Autodesk Inventor part; units mm, degrees
(part 2 of 2)
sketch "Boceto5" plane through (0, 0, 0) normal (0, 0, 1) x (1, 0, 0)
  line L0 (-116.2875, 14.8964) -> (-116.2875, 0.0237) projected
  line L1 (-116.2875, 7.46) -> (97.4125, 7.46) construction
  line L2 (97.4125, 0.0237) -> (97.4125, 14.8964) projected
  line L3 (88.5625, 9.96) -> (-107.4375, 9.96) projected
  line L4 (88.6375, 9.8301) -> (88.5625, 9.96) projected
  line L5 (-107.5125, 5.09) -> (-107.4375, 4.96) projected
  line L6 (-107.4375, 4.96) -> (88.5625, 4.96) projected
  line L7 (88.5625, 4.96) -> (88.6375, 5.09) projected
  line L8 (88.6375, 5.09) -> (97.4125, 0.0237) projected
  line L9 (97.4125, 0.0237) -> (97.4125, 14.8964) projected
  line L10 (97.4125, 14.8964) -> (88.6375, 9.8301) projected
  line L11 (88.6375, 9.8301) -> (88.5625, 9.96) projected
  line L12 (88.5625, 9.96) -> (-107.4375, 9.96) projected
  line L13 (-107.4375, 9.96) -> (-107.5125, 9.8301) projected
  line L14 (-107.5125, 9.8301) -> (-116.2875, 14.8964) projected
  line L15 (-116.2875, 14.8964) -> (-116.2875, 0.0237) projected
  line L16 (-116.2875, 0.0237) -> (-107.5125, 5.09) projected
  line L17 (88.5625, 9.96) -> (88.6375, 9.8301)
  line L18 (88.6375, 9.8301) -> (88.5625, 9.7868)
  line L19 (88.5625, 9.7868) -> (88.5625, 9.96)
  line L20 (-9.4375, 28.9561) -> (-9.4375, -11.7767) construction
  line L21 (97.4125, 14.8964) -> (88.6375, 9.8301) projected
  line L22 (88.6375, 5.09) -> (88.5625, 4.96)
  line L23 (88.6375, 5.09) -> (88.5625, 4.96)
  line L24 (88.5625, 4.96) -> (88.6375, 5.09)
  line L25 (88.6375, 5.09) -> (88.5625, 5.1333)
  line L26 (88.5625, 5.1333) -> (88.5625, 4.96)
  line L27 (-107.5125, 9.8301) -> (-107.4375, 9.96)
  line L28 (-107.4375, 4.96) -> (-107.5125, 5.09)
  line L29 (-107.5125, 9.8301) -> (-107.4375, 9.96)
  line L30 (-107.4375, 9.96) -> (-107.5125, 9.8301)
  line L31 (-107.5125, 9.8301) -> (-107.4375, 9.7868)
  line L32 (-107.4375, 9.7868) -> (-107.4375, 9.96)
  line L33 (-107.5125, 5.09) -> (-107.4375, 4.96)
  line L34 (-107.4375, 5.1333) -> (-107.4375, 4.96)
  line L35 (-107.5125, 5.09) -> (-107.4375, 4.96)
  line L36 (-107.4375, 4.96) -> (-107.5125, 5.09)
  line L37 (-107.5125, 5.09) -> (-107.4375, 5.1333)
  point P0 (0, 0)
  point P1 (-9.4375, 7.46)
  constraints: 42 end point, 19 symmetric about line, 3 midpoint, 2 vertical, 1 collinear, 1 point on line
extrude "Extrusión4" cut sketch "Boceto5" against normal through all contours L13 L32 L31 | L37 L34 L5 | L4 L18 L19 | L26 L25 L7
chamfer "Chaflán1" distance 1 angle 45 3 edges at (92.9875, 12.3416, -170) (97.4125, 7.46, -170) (92.9875, 2.5785, -170)
chamfer "Chaflán2" distance 1 angle 45 3 edges at (-111.8625, 12.3416, -170) (-116.2875, 7.46, -170) (-111.8625, 2.5785, -170)
fillet "Empalme1" radius 0.5 4 edges at (-116.2875, 14.8964, -84.5) (-116.2875, 0.0237, -84.5) (97.4125, 14.8964, -84.5) (97.4125, 0.0237, -84.5)
equation "\"d3\" = L_base"
equation "\"d14\" = Font"
equation "\"d16\" = d15"
equation "\"L_base\" = 180"
equation "\"W_Pi\" = 64.5"
equation "\"L_Pi\" = 93"
equation "\"Font\" = 36"
